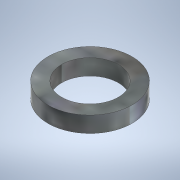
# Autodesk Inventor part: подш
Saved by Autodesk Inventor 2022 (Build 260153000, 153)
## iProperties
Created: 2022-12-27
Part Number: подш
Material: Типовые
Document SubType Name: Modeling
Designer: Pavel
Density: 1 g/cm^3
Appearance: По умолчанию
Author: Pavel
Autodesk Inventor part; units mm, degrees
ref_plane "YZ Plane" through (0, 0, 0) normal (1, 0, 0) x (0, 1, 0)
ref_plane "XZ Plane" through (0, 0, 0) normal (0, 1, 0) x (-1, 0, 0)
ref_plane "XY Plane" through (0, 0, 0) normal (0, 0, 1) x (1, 0, 0)
sketch "Эскиз1" plane through (0, 0, 0) normal (0, 1, 0) x (-1, 0, 0)
  circle A0 centre (0, 0) radius 18.5
  circle A1 centre (0, 0) radius 12.5
  dimension "d0" = 37
  dimension "d1" = 6
  constraints: 2 centre point, 2 coincident
  measures "d0" diameter of A0
  measures "d1" radial gap between concentric circles of A0 A1
extrude "Выдавливание1" add sketch "Эскиз1" along normal blind 7
